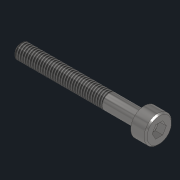
# Autodesk Inventor part: CB3-25
Saved by Autodesk Inventor 2021 (Build 250183000, 183)
## iProperties
Category: PARTsolutions
Company: MISUMI
Part Number: CB3-25
Material: 鋼、炭素鋼
Catalog Web Link: www.cadenas.de
Description: CB-Hexagon Socket Head Cap Screws
Vendor: MISUMI
Document SubType Name: Modeling
Designer: partserver
Manufacturer: MISUMI
Mass: 1.86956 g
Surface Area: 3.43168 cm^2
Volume: 0.238161 cm^3
Density: 7.85 g/cm^3
Appearance: 半つや出し
PSOL_IDENT_0: {$CADENAS_DATA\23d-libs\misumi\metric\27_screws_nuts\cb_fa.prj},150 {VTYP=3D},{NB=CB3-25},{LINA=CB3-
PSOL_IDENT_1: 25},{NN=CB},{DATE=30.06.2021 13:09:25},{GEOMDATE=17.02.2014 00:00:00},{VERSION=},{LINEID=60},{WBVAR=
PSOL_IDENT_2: L},{WBNUMERIC=L}  {NB=CB3-25},{LINA=CB3-25},{KT=DUMMY},{PN=CB3-25},{MAT=4137 Steel},{HARD=38~43HRC},
PSOL_IDENT_3: {ST=Black Oxide},{M=3},{L=25},{LL=18},{L1=18},{TYPE=CB},{M1=3.000},{L0=5,6,8,10,12,14,15,16,18,20,22
PSOL_IDENT_4: ,25,30,35,40,45,50,55},{NDM=3},{KDM=2.385665},{MP=3x0.5},{P=0.5},{A=5.5},{E=3.0},{B=2.5},{V=0.3}
NB: CB3-25
NN: CB
NT: Hexagon Socket Head Cap Screws
NBSYN: $PN.
LINA: CB3-25
CATALOG: Misumi
PN: CB3-25
MAT: 4137 Steel
HARD: 38~43HRC
ST: Black Oxide
M: 3
L: 25
LL: 18
MP: 3x0.5
A: 5.5
E: 3
B: 2.5
SUPPLIER: MISUMI
ARTICLENO: CB3-25
BOMINFO: CB3-25
CREATOR: CADENAS GmbH
Title: CB3-25
Author: Cadenas PARTsolutions
Comments: Hexagon Socket Head Cap Screws
Autodesk Inventor part; units mm, degrees
sketch "Sketch_2" plane through (0, 0, 0) normal (0, 0, 1) x (1, 0, 0)
  line L0 (25, 0) -> (-3, 0)
  line L1 (-3, 0) -> (-3, 2.45)
  line L2 (-3, 2.45) -> (-2.7, 2.75)
  line L3 (-2.7, 2.75) -> (0, 2.75)
  line L4 (0, 2.75) -> (0, 1.5)
  line L5 (0, 1.5) -> (24.6935, 1.5)
  line L6 (24.6935, 1.5) -> (25, 1.1935)
  line L7 (25, 1.1935) -> (25, 0)
  line L8 (25, 0) -> (-3, 0)
  constraints: 18 end point
revolve "Revolution1" add sketch "Sketch_2" angle 360 about axis through (25, 0, 0) along (1, 0, 0)
thread "Thread1" size "M3x0.5" class "6g" standard "ISO Metric profile" length 17.6935
sketch "Sketch2" plane through (-3, 0, 0) normal (-1, 0, 0) x (0, 0, 1)
  point P0 (0, 0)
hole "Hole1" at (-3, 0, 0) direction (1, 0, 0) diameter 2.5 depth 1.5 tip angle 150
sketch "Sketch_3" plane through (-3, 0, 0) normal (1, 0, 0) x (0, 0, -1)
  line L0 (-1.25, -0.7217) -> (0, -1.4434)
  line L1 (0, -1.4434) -> (1.25, -0.7217)
  line L2 (1.25, -0.7217) -> (1.25, 0.7217)
  line L3 (1.25, 0.7217) -> (0, 1.4434)
  line L4 (0, 1.4434) -> (-1.25, 0.7217)
  line L5 (-1.25, 0.7217) -> (-1.25, -0.7217)
  constraints: 12 end point
extrude "Extrusion1" cut sketch "Sketch_3" along normal blind 1.5
ref_plane "bolt_to_nut_XY" through (25, 0, 0) normal (1, 0, 0) x (0, 0, -1)
ref_plane "bolt_to_nut_YZ" through (25, 0, 0) normal (0, 0, -1) x (0, 1, 0)
ref_plane "bolt_to_nut_ZX" through (25, 0, 0) normal (0, 1, 0) x (1, 0, 0)
ref_plane "screw1_XY" through (0, 0, 0) normal (1, 0, 0) x (0, 0, -1)
ref_plane "screw1_YZ" through (0, 0, 0) normal (0, 0, -1) x (0, 1, 0)
ref_plane "screw1_ZX" through (0, 0, 0) normal (0, 1, 0) x (1, 0, 0)
body "Solid1"
